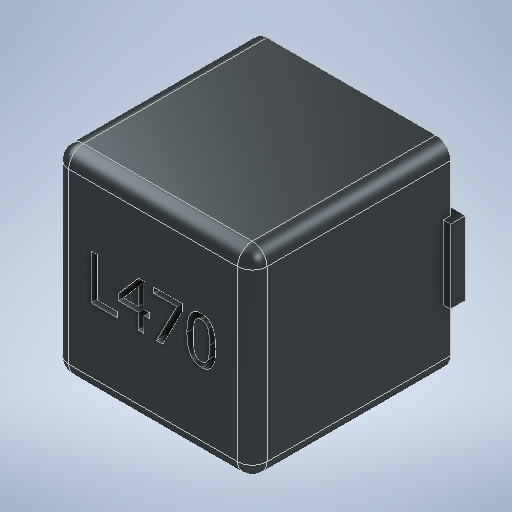
# Autodesk Inventor part: SINC1313-470_L470_SMD
Saved by Autodesk Inventor 2025.1 (Build 291241000, 241)
## iProperties
Created: 2024-05-16
Part Number: SINC1313-470_L470_SMD
Material: ABS Plastic
Document SubType Name: Modeling
Designer: Roman Suk
Density: 1.06 g/cm^3
Appearance: Železo – šedé
MASSSFP: 400 g
SFP: 4HR
Author: Roman Suk
## iProperties of the stored document SINC1313-470_L470_SMD_3DPrint.ipt
Created: 2024-05-16
Part Number: SINC1313-470_L470_SMD_3DPrint
Material: Generic
Document SubType Name: Modeling
Designer: Roman Suk
Density: 1 g/cm^3
Appearance: Default
Author: Roman Suk
Autodesk Inventor part; units mm, degrees
ref_plane "YZ Plane" through (0, 0, 0) normal (1, 0, 0) x (0, 1, 0)
ref_plane "XZ Plane" through (0, 0, 0) normal (0, 1, 0) x (-1, 0, 0)
ref_plane "XY Plane" through (0, 0, 0) normal (0, 0, 1) x (1, 0, 0)
sketch "Sketch2" plane through (0, 0, 0) normal (0, 0, 1) x (1, 0, 0)
  line L0 (-6.75, -6.75) -> (6.75, -6.75)
  line L1 (6.75, -6.75) -> (6.75, 6.75)
  line L2 (6.75, 6.75) -> (-6.75, 6.75)
  line L3 (-6.75, 6.75) -> (-6.75, -6.75)
  line L4 (-6.75, -6.75) -> (6.75, 6.75) construction
  line L5 (6.75, -6.75) -> (-6.75, 6.75) construction
  line L6 (-6.75, -6.75) -> (6.75, -6.75) construction
  line L7 (6.75, -6.75) -> (6.75, -2.5) construction
  line L8 (6.75, -2.5) -> (-6.75, -2.5) construction
  line L9 (-6.75, -2.5) -> (-6.75, -6.75) construction
  line L10 (-7.25, -2.5) -> (7.25, -2.5)
  line L11 (7.25, -2.5) -> (7.25, 2.5)
  line L12 (7.25, 2.5) -> (-7.25, 2.5)
  line L13 (-7.25, 2.5) -> (-7.25, -2.5)
  line L14 (-7.25, 2.5) -> (-5.25, 2.5)
  line L15 (-5.25, 2.5) -> (-5.25, -2.5)
  line L16 (-5.25, -2.5) -> (-7.25, -2.5)
  line L17 (-7.25, -2.5) -> (-7.25, 2.5)
  line L18 (7.25, 2.5) -> (5.25, 2.5)
  line L19 (5.25, 2.5) -> (5.25, -2.5)
  line L20 (5.25, -2.5) -> (7.25, -2.5)
  line L21 (7.25, -2.5) -> (7.25, 2.5)
  line L22 (4.25, -4.25) -> (-4.25, -4.25)
  line L23 (-4.25, -4.25) -> (-4.25, 4.25)
  line L24 (-4.25, 4.25) -> (4.25, 4.25)
  line L25 (4.25, 4.25) -> (4.25, -4.25)
  line L26 (4.25, -4.25) -> (-4.25, 4.25) construction
  line L27 (-4.25, -4.25) -> (4.25, 4.25) construction
  point P0 (0, 0)
  point P1 (0, -2.5)
  point P2 (-6.75, 2.5)
  point P3 (6.75, -2.5)
  point P4 (6.75, 2.5)
  dimension "d2" = 13.5
  dimension "d4" = 4.25
  dimension "d5" = 5
  dimension "d6" = 0.5
  dimension "d7" = 0.5
  dimension "d8" = 2
  dimension "d9" = 2
  dimension "d16" = 8.5
  constraints: 56 end point, 12 parallel, 8 perpendicular, 6 horizontal, 5 midpoint, 3 point on line, 1 horizontal alignment
  measures "d2" distance of L2.end L1.end
  measures "d4" distance between parallel lines of L0 L8
  measures "d5" distance between parallel lines of L12 L10
  measures "d6" distance between parallel lines of L3 L13
  measures "d7" distance between parallel lines of L1 L11
  measures "d8" distance of L15.end L16.end
  measures "d9" distance of L20.end L19.end
  measures "d16" distance of L23.end L24.end
extrude "Extrusion2" add sketch "Sketch2" along normal blind 13.5 contours L3 L10 L23 L22 L25 L1 L0 | L3 L12 L15 L10 | L10 L19 L12 L1 | L3 L2 L1 L12 L25 L24 L23 | L15 L12 L23 L10 | L10 L25 L12 L19 | L23 L12 L25 L10 | L10 L25 L22 L23 | L23 L24 L25 L12
extrude "Extrusion3" add sketch "Sketch2" against normal blind 0.5 contours L3 L12 L15 L10 | L10 L19 L12 L1
extrude "Extrusion4" add sketch "Sketch2" along normal mid plane 1 contours L10 L13 L12 L3 | L1 L12 L11 L10
extrude "Extrusion5" cut sketch "Sketch2" along normal blind 10 contours L23 L12 L25 L10 | L10 L25 L22 L23 | L23 L24 L25 L12
sketch "Sketch3" plane through (0, 0, 13.5) normal (0, 0, 1) x (1, 0, 0)
  line L0 (-4.532, 1.7426) -> (3.9775, 1.7426) construction
  line L1 (3.9775, 1.7426) -> (3.9775, -2.8625) construction
  line L2 (3.9775, -2.8625) -> (-4.532, -2.8625) construction
  line L3 (-4.532, -2.8625) -> (-4.532, 1.7426) construction
  line L4 (-2.4572, -1.3672) -> (-4.2232, -1.3672)
  line L5 (-4.2232, -1.3672) -> (-4.2232, 1.6808)
  line L6 (-4.2232, 1.6808) -> (-3.8182, 1.6808)
  line L7 (-3.8182, 1.6808) -> (-3.8182, -1.0065)
  line L8 (-3.8182, -1.0065) -> (-2.4572, -1.0065)
  line L9 (-2.4572, -1.0065) -> (-2.4572, -1.3672)
  line L10 (-0.2638, -0.3199) -> (-0.6269, -0.3199)
  line L11 (-0.6269, -0.3199) -> (-0.6269, -1.3672)
  line L12 (-0.6269, -1.3672) -> (-1.0196, -1.3672)
  line L13 (-1.0196, -1.3672) -> (-1.0196, -0.3199)
  line L14 (-1.0196, -0.3199) -> (-2.3658, -0.3199)
  line L15 (-2.3658, -0.3199) -> (-2.3658, 0.1099)
  line L16 (-2.3658, 0.1099) -> (-1.0023, 1.6808)
  line L17 (-1.0023, 1.6808) -> (-0.6269, 1.6808)
  line L18 (-0.6269, 1.6808) -> (-0.6269, 0.0086)
  line L19 (-0.6269, 0.0086) -> (-0.2638, 0.0086)
  line L20 (-0.2638, 0.0086) -> (-0.2638, -0.3199)
  line L21 (-1.0196, 0.0086) -> (-1.0196, 1.1992)
  line L22 (-1.0196, 1.1992) -> (-2.0447, 0.0086)
  line L23 (-2.0447, 0.0086) -> (-1.0196, 0.0086)
  line L24 (1.9765, 1.2239) -> (0.6575, -1.3672)
  line L25 (0.6575, -1.3672) -> (0.2228, -1.3672)
  line L26 (0.2228, -1.3672) -> (1.6159, 1.3227)
  line L27 (1.6159, 1.3227) -> (0.0425, 1.3227)
  line L28 (0.0425, 1.3227) -> (0.0425, 1.6808)
  line L29 (0.0425, 1.6808) -> (1.9765, 1.6808)
  line L30 (1.9765, 1.6808) -> (1.9765, 1.2239)
  spline S0 degree 2 poles (4.2464, 0.1568) (4.2464, -0.6632) (3.7697, -1.4314) (3.2733, -1.4314) knots 0 0 0 1 2 2 2
  spline S1 degree 2 poles (3.2733, -1.4314) (2.7694, -1.4314) (2.2976, -0.6484) (2.2976, 0.1544) knots 0 0 0 1 2 2 2
  spline S2 degree 2 poles (2.2976, 0.1544) (2.2976, 0.9794) (2.7743, 1.7426) (3.2733, 1.7426) knots 0 0 0 1 2 2 2
  spline S3 degree 2 poles (3.2733, 1.7426) (3.7747, 1.7426) (4.2464, 0.9522) (4.2464, 0.1568) knots 0 0 0 1 2 2 2
  spline S4 degree 2 poles (3.7228, -0.7719) (3.7821, -0.6212) (3.8315, -0.1569) (3.8315, 0.1568) knots 0 0 0 1 2 2 2
  spline S5 degree 2 poles (3.8315, 0.1568) (3.8315, 0.4705) (3.7821, 0.9324) (3.7203, 1.088) knots 0 0 0 1 2 2 2
  spline S6 degree 2 poles (3.7203, 1.088) (3.6586, 1.2436) (3.4437, 1.4042) (3.2733, 1.4042) knots 0 0 0 1 2 2 2
  spline S7 degree 2 poles (3.2733, 1.4042) (3.1028, 1.4042) (2.883, 1.2436) (2.8188, 1.0831) knots 0 0 0 1 2 2 2
  spline S8 degree 2 poles (2.8188, 1.0831) (2.757, 0.9275) (2.7126, 0.4532) (2.7126, 0.1544) knots 0 0 0 1 2 2 2
  spline S9 degree 2 poles (2.7126, 0.1544) (2.7126, -0.1667) (2.7521, -0.5965) (2.8163, -0.7645) knots 0 0 0 1 2 2 2
  spline S10 degree 2 poles (2.8163, -0.7645) (2.8756, -0.9226) (3.0954, -1.093) (3.2733, -1.093) knots 0 0 0 1 2 2 2
  spline S11 degree 2 poles (3.2733, -1.093) (3.4412, -1.093) (3.6611, -0.9324) (3.7228, -0.7719) knots 0 0 0 1 2 2 2
  point P0 (0, 0)
  constraints: 2 other
fillet "Fillet1" radius 1 8 edges at (0, 6.75, 13.5) (-6.75, 0, 13.5) (0, -6.75, 13.5) (6.75, 0, 13.5) (-6.75, 6.75, 6.75) (-6.75, -6.75, 6.75) (6.75, 6.75, 6.75) (6.75, -6.75, 6.75)
extrude "Extrusion7" cut sketch "Sketch3" against normal blind 1
body "Solid2"
